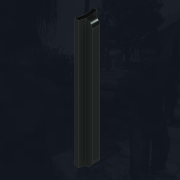
# Autodesk Inventor part: Grip
Saved by Autodesk Inventor 2021 (Build 250183000, 183)
## iProperties
Created: 2021-01-08
Part Number: Grip
Material: Generic
Document SubType Name: Modeling
Designer: Alex
Density: 1 g/cm^3
Appearance: Default
Author: Alex
Autodesk Inventor part; units mm, degrees
ref_plane "YZ Plane" through (0, 0, 0) normal (1, 0, 0) x (0, 1, 0)
ref_plane "XZ Plane" through (0, 0, 0) normal (0, 1, 0) x (-1, 0, 0)
sketch "Sketch1" plane through (0, 0, 0) normal (0, 1, 0) x (-1, 0, 0)
  arc A0 (-1.337, 0) -> (0, -5.9706) centre (12.663, 0) ccw
  line L0 (-1.337, 0) -> (0, 0)
  line L1 (0, -5.9706) -> (-2.6226, -6.213)
  line L2 (0, -5.9706) -> (5.1195, -5.9706) construction
  line L3 (0, 5.9706) -> (-2.6226, 6.213)
  line L4 (0, 5.9706) -> (2.6337, 5.9706) construction
  arc A1 (0, 5.9706) -> (-1.337, 0) centre (12.663, 0) ccw
  line L5 (-3.6462, -2.502) -> (-3.837, -2.502)
  line L6 (-3.6462, 2.502) -> (-3.837, 2.502)
  line L7 (-3.837, -2.502) -> (-8.337, -2.502)
  line L8 (-8.337, -2.502) -> (-8.337, 2.502)
  line L9 (-8.337, 2.502) -> (-3.837, 2.502)
  arc A2 (-2.6226, 6.213) -> (-3.6462, 2.502) centre (12.663, 0) ccw
  arc A3 (-3.6462, -2.502) -> (-2.6226, -6.213) centre (12.663, 0) ccw
  dimension "d2" = 174.72
  dimension "d3" = 174.72
  dimension "d7" = 4.5
  constraints: 20 end point, 8 point on circle, 4 centre point, 3 horizontal, 1 coincident, 1 equal length, 1 perpendicular
  measures "d2" angle of L1 L2
  measures "d3" angle of L4 L3
  measures "d7" distance of L5.end L7.end
extrude "Extrusion1" add sketch "Sketch1" along normal blind 85.8
fillet "Fillet1" radius 4.5 2 edges at (8.337, 85.8, 0) (8.337, 0, 0)
ref_plane "Work Plane1" through (3.837, 85.8, -2.502) normal (-1, 0, 0) x (0, -1, 0)
sketch "Sketch2" plane through (3.837, 85.8, -2.502) normal (-1, 0, 0) x (0, -1, 0)
  line L0 (0, 0) -> (0, 5.004) projected
  line L1 (0, 2.502) -> (15, 2.502) construction
  line L2 (85.8, 5.004) -> (85.8, 0) projected
  line L3 (85.8, 2.502) -> (70.8, 2.502) construction
  circle A0 centre (15, 2.502) radius 1.5
  line L4 (70.8, 2.502) -> (70.9, 2.502) construction
  circle A1 centre (70.9, 2.502) radius 1.5
  line L5 (70.9, 2.502) -> (71.1, 2.502) construction
  line L6 (71.1, 2.502) -> (71.1, 4.6181) construction
  dimension "d11" = 15
  dimension "d13" = 3
  dimension "d23" = 0.2
  constraints: 10 end point, 3 coincident, 2 centre point, 2 horizontal, 2 perpendicular, 1 midpoint, 1 point on line
  measures "d11" distance of L1.start L1.end
  measures "d13" diameter of A0
  measures "d23" distance of L5.start L5.end
extrude "Extrusion2" cut sketch "Sketch2" along normal blind 7 contours A0
extrude "Extrusion3" cut sketch "Sketch2" along normal up to surface contours A1
body "Solid1"
